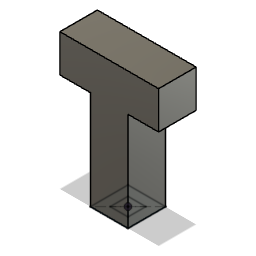
T-Griff v2 (Autodesk Fusion 360 design; units mm, degrees)
Autodesk Fusion 360 part; units mm, degrees
sketch "Skizze1" plane through (0, 0, 0) normal (0, 1, 0) x (1, 0, 0)
  line L0 (9.5, 9.5) -> (-9.5, 9.5)
  line L1 (-9.5, 9.5) -> (-9.5, -9.5)
  line L2 (-9.5, -9.5) -> (9.5, -9.5)
  line L3 (9.5, -9.5) -> (9.5, 9.5)
  line L4 (9.5, 9.5) -> (-9.5, -9.5) construction
  line L5 (-9.5, 9.5) -> (9.5, -9.5) construction
  line L6 (4.5, 4.5) -> (-4.5, 4.5)
  line L7 (-4.5, 4.5) -> (-4.5, -4.5)
  line L8 (-4.5, -4.5) -> (4.5, -4.5)
  line L9 (4.5, -4.5) -> (4.5, 4.5)
  line L10 (4.5, 4.5) -> (-4.5, -4.5) construction
  line L11 (-4.5, 4.5) -> (4.5, -4.5) construction
  dimension "d1" = 19
  dimension "d2" = 19
  dimension "d3" = 9
  dimension "d4" = 9
  constraint horizontal L0
  constraint perpendicular L0 L1
  constraint parallel L0 L2
  constraint parallel L1 L3
  constraint coincident L4 origin
  constraint coincident L5 origin
  constraint horizontal L6
  constraint perpendicular L6 L7
  constraint parallel L6 L8
  constraint parallel L7 L9
  constraint coincident L10 origin
  constraint coincident L11 origin
  measures "d1" distance of L1.end L2.end
  measures "d2" distance of L0.end L1.end
  measures "d3" distance of L7.end L8.end
  measures "d4" distance of L6.end L7.end
extrude "Extrusion1" add sketch "Skizze1" along normal blind 50 contours L0 L1 L2 L3 | L6 L7 L8 L9 makes body 1
ref_plane "Arbeitsebene1" through (0, 25, 0) normal (1, 0, 0) x (0, 0, -1)
sketch "Skizze2" plane through (0, 25, 0) normal (1, 0, 0) x (0, 0, -1)
  line L0 (-9.5, 25) -> (9.5, 25)
  line L1 (9.5, 25) -> (9.5, 44)
  line L2 (9.5, 44) -> (-9.5, 44)
  line L3 (-9.5, 44) -> (-9.5, 25)
  dimension "d8" = 19
  dimension "d9" = 19
  constraint horizontal L0
  constraint vertical L1
  constraint horizontal L2
  constraint vertical L3
  measures "d8" distance of L0.start L0.end
  measures "d9" distance of L0.start L2.end
extrude "Extrusion2" add sketch "Skizze2" along normal mid plane 50 bodies 1
extrude "Extrusion3" cut sketch "Skizze1" along normal blind 10 contours L6 L7 L8 L9 bodies 1
copy_body "Körper->Berechn1" bodies 1 removing the originals makes body 2 in component "T-Griff"
component "T-Griff" placed x (1, 0, 0) y (0, 1, 0) z (0, 0, 1) at (0, 0, 0)
